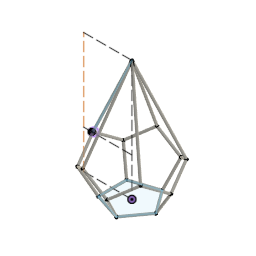
Deco (Autodesk Fusion 360 design; units mm, degrees)
Autodesk Fusion 360 part; units mm, degrees
sketch "Sketch1" plane through (0, 0, 0) normal (0, 0, 1) x (1, 0, 0) in component "Base"
  line L0 (100, 0) -> (30.901699, 95.105652)
  line L1 (30.901699, 95.105652) -> (-80.901699, 58.778525)
  line L2 (-80.901699, 58.778525) -> (-80.901699, -58.778525)
  line L3 (-80.901699, -58.778525) -> (30.901699, -95.105652)
  line L4 (30.901699, -95.105652) -> (100, 0)
  circle A0 centre (0, 0) radius 5
  dimension "d1" = 100
  dimension "d10" = 10
  constraint coincident A0.centre origin
  measures "d1" distance of L0.start A0.centre
  measures "d10" diameter of A0
pipe "Pipe1" add diameter 10 path "Sketch1" along L4 L0 L1 L2 L3 makes body 1 in component "Base"
copy_body "CopyPasteBodies1" bodies 1 makes body 2 in component "Base"
move_body "Move1" bodies 2 to x (0.80901699, -0.58778525, 0) y (-0.58778525, -0.80901699, 0) z (0, 0, -1) at (-50, -153.884177, 0) in component "Base"
move_body "Move2" bodies 2 to x (0.94721352, -0.16246008, -0.27639333) y (-0.16246008, 0.49999928, -0.85065119) z (0.27639333, 0.85065119, 0.4472128) at (-13.81968, -42.532602, -72.360712) in component "Base"
pattern_circular "C-Pattern1" count 5 over 360 about axis through (0, 0, 1.75) along (0, 0, 1) of bodies 2 makes body 3 at (80.354874, -34.163149, -2.73241) makes body 4 at (57.322107, 65.865033, -2.73241) makes body 5 at (-44.927863, 74.869978, -2.73241) makes body 6 at (-85.089054, -19.592842, -2.73241) in component "Base"
sketch "Sketch4" plane through (0, 0, 0) normal (0, 1, 0) x (1, 0, 0) in component "Base"
  line L0 (0, 0) -> (-200, 0) construction
  line L1 (-200, 0) -> (-200, -500) construction
  line L2 (-200, -500) -> (0, -500) construction
  line L3 (0, -500) -> (0, 0) construction
  line L4 (-200, -159.567407) -> (0, -159.567407) construction
  line L5 (-166.275392, -159.567407) -> (-160.162384, -159.567407)
  line L6 (-163.218888, -159.567407) -> (0, -500)
  point P0 (-166.275392, -159.567407)
  point P1 (-157.331116, -164.039535)
  dimension "d13" = 500
  constraint coincident L0.start L3.end
  constraint horizontal L0
  constraint perpendicular L0 L1
  constraint perpendicular L1 L2
  constraint perpendicular L0 L3
  constraint perpendicular L3 L4
  constraint parallel L4 L5
  measures "d13" distance of L2.end L0.start
pipe "Pipe2" add diameter 10 path "Sketch4" along L6 separate body makes body 7 in component "Base"
pattern_circular "C-Pattern2" count 5 over 360 about axis through (0, 0, 500) along (0, 0, -1) of bodies 7 makes body 8 at (-28.764264, 104.643032, 272.851957) makes body 9 at (87.20456, 59.30514, 271.412937) makes body 10 at (89.788259, -59.319342, 272.419103) makes body 11 at (-28.764264, -104.643032, 272.851957) in component "Base"
combine "Combine1" operation add target body 1 tool bodies 4 7 6 2 3 5 8 9 10 11 in component "Base"
component "Base" placed x (1, 0, 0) y (0, 1, 0) z (0, 0, 1) at (0, 0, 0)
equation "d1 = PentagonSIze"
equation "d4 = TubeSize"
equation "PentagonSIze = 100 mm"
equation "TubeSize = 10 mm"
equation "d13 = Height"
equation "d16 = TubeSize"
equation "Height = 500 mm"
